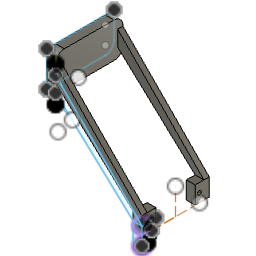
vocalink-mount (Autodesk Fusion 360 design; units mm, degrees)
Autodesk Fusion 360 part; units mm, degrees
sketch "Sketch1" plane through (0, 0, 0) normal (1, 0, 0) x (0, 1, 0)
  line L0 (5, 75) -> (33.358, 75)
  line L1 (38.358, 70) -> (38.358, 60)
  line L2 (33.358, 55) -> (5, 55)
  line L3 (0, 60) -> (0, 70)
  arc A0 (5, 75) -> (0, 70) centre (5, 70) ccw
  arc A1 (38.358, 70) -> (33.358, 75) centre (33.358, 70) ccw
  arc A2 (33.358, 55) -> (38.358, 60) centre (33.358, 60) ccw
  arc A3 (0, 60) -> (5, 55) centre (5, 60) ccw
  point P0 (0, 75)
  point P1 (38.358, 75)
  point P2 (0, 55)
  dimension "d1" = 38.358
  dimension "d2" = 20
  dimension "d3" = 5
  constraint horizontal L0
  constraint vertical L1
  constraint horizontal L2
  constraint vertical L3
  constraint coincident P0 L0
  constraint coincident P0 L3
  constraint tangent L0 A0
  constraint tangent L3 A0
  constraint coincident P1 L0
  constraint coincident P1 L1
  constraint tangent L0 A1
  constraint tangent L1 A1
  constraint equal A0 A1
  constraint tangent L1 A2
  constraint tangent L2 A2
  constraint equal A0 A2
  constraint coincident P2 L2
  constraint coincident P2 L3
  constraint tangent L2 A3
  constraint tangent L3 A3
  constraint equal A0 A3
  measures "d1" distance of P0 P1
  measures "d2" distance of P0 P2
  measures "d3" radius of A0
sketch "Sketch2" plane through (0, 0, 0) normal (0, 1, 0) x (1, 0, 0)
  line L0 (5, -50) -> (5, -70)
  line L1 (5, -64.4916) -> (54.177, -14.6758)
  line L2 (54.177, -14.6758) -> (49.177, -14.6758)
  line L3 (49.177, -14.6758) -> (49.177, -6.6758)
  line L4 (51.177, -4.6758) -> (52.177, -4.6758)
  line L5 (54.177, -6.6758) -> (54.177, -14.6758)
  arc A0 (8.724, -60.7193) -> (5, -70) centre (17.919, -69.7964) ccw
  arc A1 (5, -50) -> (14.5871, -47.156) centre (6.4053, -37.156) ccw
  line L6 (5, -55.6374) -> (49.177, -14.6758)
  line L7 (51.177, -4.6758) -> (49.177, -4.6758)
  line L8 (49.177, -4.6758) -> (49.177, -6.6758)
  line L9 (52.177, -4.6758) -> (54.177, -4.6758)
  line L10 (54.177, -4.6758) -> (54.177, -6.6758)
  point P0 (54.177, -4.6758)
  dimension "d6" = 70
  dimension "d8" = 5
  dimension "d9" = 10
  dimension "d12" = 10
  dimension "d13" = 10
  constraint coincident L0 L1.start
  constraint horizontal L2
  constraint vertical L3
  constraint horizontal L4
  constraint vertical L5
  constraint tangent L1 A0
  constraint coincident L1 A0.start
  constraint coincident L0.end A0.end
  constraint coincident L0.start A1.start
  constraint coincident P0 L4
  constraint coincident P0 L5
  constraint coincident L0 L6.start
  constraint horizontal L7
  constraint vertical L8
  constraint horizontal L9
  constraint vertical L10
  measures "d6" distance of L1.start L1.end
  measures "d8" distance of L1.end L2.end
  measures "d9" distance of L1.end P0
  measures "d12" distance of L0.end A0.start
  measures "d13" distance of L0.start A1.end
sketch "Sketch4" plane through (54.177, 0, 0) normal (1, 0, 0) x (0, 1, 0)
extrude "Extrude7" add sketch "Sketch2" along normal blind 3 contours L0 L1 L2 L6 | L2 L3 L4 L5 L7 L8 L9 L10 makes body 1
sketch "Sketch5" plane through (54.177, 0, 0) normal (1, 0, 0) x (0, 1, 0)
  line L0 (3, 4.6758) -> (3, 14.6758)
  line L1 (8, 14.6758) -> (8, 4.6758)
  line L2 (3, 4.6758) -> (3, 14.6758)
  line L3 (8, 4.6758) -> (8, 14.6758) construction
  line L4 (3, 14.6758) -> (8, 14.6758)
  line L5 (3, 4.6758) -> (8, 4.6758)
  line L6 (0, 4.6758) -> (0, 14.6758) construction
  circle A0 centre (5.5416, 9.5926) radius 1.065
  line L7 (5.5416, 9.5926) -> (32.8166, 9.5926) construction
  line L8 (5.5416, 9.5926) -> (19.1791, 9.5926) construction
  line L9 (19.1791, 9.5926) -> (19.1791, 24.5926) construction
  point P0 (8, 14.6758)
  dimension "d29" = 10
  dimension "d36" = 2.13
  dimension "d39" = 27.275
  dimension "d40" = 13.6375
  dimension "d41" = 15
  constraint vertical L1
  constraint vertical L2
  constraint coincident L0.end L2.end
  constraint coincident P0 L1
  constraint coincident P0 L1.start
  constraint parallel L1 L3
  constraint perpendicular L1 L4
  constraint coincident L0.start L2.start
  constraint perpendicular L1 L5
  constraint horizontal L7
  constraint coincident A0.centre L7.start
  constraint horizontal L8
  constraint perpendicular L7 L9
  measures "d29" distance of L0.end L0.start
  measures "d36" diameter of A0
  measures "d39" distance of A0.centre L7.end
  measures "d40" distance of A0.centre L8.end
  measures "d41" distance of L8.end L9.end
extrude "Extrude8" add sketch "Sketch5" against normal blind 5 contours L0 L1 L2 L4 L5 | A0 bodies 1
extrude "Extrude9" add sketch "Sketch1" along normal blind 5 separate body makes body 2
extrude "Extrude10" cut sketch "Sketch5" against normal blind 5 contours A0 bodies 1
mirror "Mirror1" about plane through (0, 0, 0) normal (0, 1, 0) of bodies 1 makes body 3
move_body "Move1" bodies 3 to x (1, 0, 0) y (0, 1, 0) z (0, 0, 1) at (0, 38, 0)
move_body "Move2" bodies 3 to x (1, 0, 0) y (0, 1, 0) z (0, 0, 1) at (0, 0.3581, 0)
move_body "Move3" bodies 3 1 to x (1, 0, 0) y (0, 1, 0) z (0, 0, 1) at (0, 0, 5)
named bodies: "Base", "Arm", "Arm (1)"
